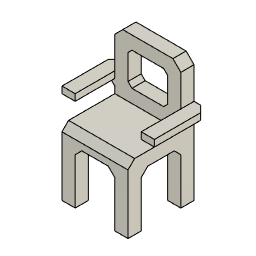
Demonstrationsmodell Kurs 3D-skrivare v3 (Autodesk Fusion 360 design; units mm, degrees)
Autodesk Fusion 360 part; units mm, degrees
sketch "Sketch1" plane through (0, 0, 0) normal (0, 0, 1) x (1, 0, 0) in component "Chair Brutaliste"
  line L0 (0, 0) -> (10, 0)
  line L1 (10, 0) -> (10, 10)
  line L2 (10, 10) -> (0, 10)
  line L3 (0, 10) -> (0, 0)
  line L4 (0, 0) -> (50, 0) construction
  line L5 (50, 0) -> (50, 50) construction
  line L6 (50, 50) -> (0, 50) construction
  line L7 (50, 0) -> (40, 0)
  line L8 (40, 0) -> (40, 10)
  line L9 (40, 10) -> (50, 10)
  line L10 (50, 10) -> (50, 0)
  line L11 (50, 50) -> (40, 50)
  line L12 (40, 50) -> (40, 40)
  line L13 (40, 40) -> (50, 40)
  line L14 (50, 40) -> (50, 50)
  line L15 (0, 50) -> (10, 50)
  line L16 (10, 50) -> (10, 40)
  line L17 (10, 40) -> (0, 40)
  line L18 (0, 40) -> (0, 50)
  dimension "d1" = 10
  dimension "d2" = 50
  constraint horizontal L0
  constraint vertical L1
  constraint horizontal L2
  constraint vertical L3
  constraint coincident L0.start L3.end
  constraint equal L1 L2
  constraint perpendicular L3 L4
  constraint perpendicular L4 L5
  constraint perpendicular L5 L6
  constraint horizontal L7
  constraint vertical L8
  constraint horizontal L9
  constraint vertical L10
  constraint horizontal L11
  constraint vertical L12
  constraint horizontal L13
  constraint vertical L14
  constraint horizontal L15
  constraint vertical L16
  constraint horizontal L17
  constraint vertical L18
  constraint equal L16 L17
  constraint equal L12 L13
  constraint equal L8 L9
  constraint equal L1 L8
  constraint equal L9 L13
  constraint equal L13 L16
  constraint equal L4 L6
  constraint equal L4 L5
  measures "d1" distance of L0.start L0.end
  measures "d2" distance of L0.start L4.end
extrude "Extrude1" add sketch "Sketch1" along normal blind 40 makes body 1 at (3.3333, 50, 13.3333) makes body 2 at (0, 6.6667, 13.3333) makes body 3 at (50, 43.3333, 13.3333) makes body 4 at (43.3333, 10, 13.3333) in component "Chair Brutaliste"
sketch "Sketch2" plane through (0, 0, 40) normal (0, 0, 1) x (-1, 0, 0) in component "Chair Brutaliste"
  line L0 (-50, -10) -> (-40, -10)
  line L1 (-40, -10) -> (-40, 0)
  line L2 (-40, 0) -> (-50, 0)
  line L3 (-50, 0) -> (-50, -10)
  line L4 (-50, -50) -> (0, -50)
  line L5 (0, -50) -> (0, 0)
  line L6 (0, 0) -> (-50, 0)
  line L7 (-50, 0) -> (-50, -50)
  constraint horizontal L4
  constraint vertical L5
  constraint horizontal L6
  constraint vertical L7
  constraint coincident L5.end L6.start
extrude "Extrude2" add sketch "Sketch2" along normal blind 10 bodies 1 2 3 4 in component "Chair Brutaliste"
sketch "Sketch3" plane through (50, 0, 0) normal (1, 0, 0) x (0, 1, 0) in component "Chair Brutaliste"
  line L0 (40, 0) -> (50, 0)
  line L1 (50, 0) -> (50, 50)
  line L2 (50, 50) -> (0, 50)
  line L3 (0, 50) -> (0, 0)
  line L4 (0, 0) -> (10, 0)
  line L5 (10, 0) -> (10, 40)
  line L6 (10, 40) -> (40, 40)
  line L7 (40, 40) -> (40, 0)
  line L8 (50, 50) -> (40, 50)
  line L9 (40, 50) -> (40, 95)
  line L10 (40, 95) -> (50, 95)
  line L11 (50, 95) -> (50, 50)
  dimension "d8" = 10
  dimension "d9" = 45
  constraint horizontal L8
  constraint vertical L9
  constraint horizontal L10
  constraint vertical L11
  constraint coincident L1.end L2.start
  measures "d8" distance of L1.end L8.end
  measures "d9" distance of L1.end L10.end
extrude "Extrude3" add sketch "Sketch3" against normal up to surface (50 mm away) contours L2 L8 L9 L10 L11 bodies 1 in component "Chair Brutaliste"
sketch "Sketch4" plane through (0, 40, 0) normal (0, -1, 0) x (1, 0, 0) in component "Chair Brutaliste"
  line L0 (0, 95) -> (0, 50)
  line L1 (0, 50) -> (50, 50)
  line L2 (50, 50) -> (50, 95)
  line L3 (50, 95) -> (0, 95)
  line L4 (10, 60) -> (40, 60)
  line L5 (40, 60) -> (40, 85)
  line L6 (40, 85) -> (10, 85)
  line L7 (10, 85) -> (10, 60)
  dimension "d13" = -10
extrude "Extrude4" cut sketch "Sketch4" against normal up to surface (10 mm away) contours L4 L5 L6 L7 bodies 1 in component "Chair Brutaliste"
chamfer "Chamfer2" distance 5 angle 45 8 edges at (10, 45, 40) (10, 5, 40) (40, 45, 40) (40, 5, 40) (5, 40, 40) (5, 10, 40) (45, 40, 40) (45, 10, 40) on bodies 1 in component "Chair Brutaliste"
chamfer "Chamfer3" distance 3 angle 45 4 edges at (40, 45, 85) (10, 45, 85) (10, 45, 60) (40, 45, 60) on bodies 1 in component "Chair Brutaliste"
chamfer "Chamfer4" distance 6 angle 45 2 edges at (50, 45, 95) (0, 45, 95) on bodies 1 in component "Chair Brutaliste"
sketch "Sketch5" plane through (50, 0, 0) normal (1, 0, 0) x (0, 1, 0) in component "Chair Brutaliste"
  line L0 (50, 89) -> (40, 89)
  line L1 (40, 89) -> (40, 50)
  line L2 (40, 50) -> (0, 50)
  line L3 (0, 50) -> (0, 0)
  line L4 (0, 0) -> (10, 0)
  line L5 (10, 0) -> (10, 35)
  line L6 (10, 35) -> (15, 40)
  line L7 (15, 40) -> (35, 40)
  line L8 (35, 40) -> (40, 35)
  line L9 (40, 35) -> (40, 0)
  line L10 (40, 0) -> (50, 0)
  line L11 (50, 0) -> (50, 89)
  line L12 (40, 50) -> (40, 60) construction
  line L13 (40, 60) -> (40, 65)
  line L14 (40, 60) -> (50, 60)
  line L15 (40, 65) -> (50, 65)
  line L16 (50, 60) -> (50, 65)
  dimension "d19" = 5
  dimension "d20" = 10
  constraint coincident L1.end L2.start
  constraint coincident L1 L12.end
  constraint perpendicular L2 L12
  constraint coincident L1 L13.end
  constraint parallel L1 L13
  constraint coincident L11 L14.end
  constraint perpendicular L11 L14
  constraint coincident L11 L15.end
  constraint perpendicular L11 L15
  measures "d19" distance of L12.end L13.end
  measures "d20" distance of L1.end L12.end
extrude "Extrude5" add sketch "Sketch5" along normal blind 10 contours L1 L11 L13 L14 L15 L16 bodies 1 in component "Chair Brutaliste"
sketch "Sketch6" plane through (0, 40, 0) normal (0, -1, 0) x (1, 0, 0) in component "Chair Brutaliste"
  line L0 (13, 85) -> (37, 85)
  line L1 (37, 85) -> (40, 82)
  line L2 (40, 82) -> (40, 63)
  line L3 (40, 63) -> (37, 60)
  line L4 (37, 60) -> (13, 60)
  line L5 (13, 60) -> (10, 63)
  line L6 (10, 63) -> (10, 82)
  line L7 (10, 82) -> (13, 85)
  line L8 (6, 95) -> (0, 89)
  line L9 (0, 89) -> (0, 50)
  line L10 (0, 50) -> (50, 50)
  line L11 (50, 50) -> (50, 60)
  line L12 (50, 60) -> (60, 60)
  line L13 (60, 60) -> (60, 65)
  line L14 (60, 65) -> (50, 65)
  line L15 (50, 65) -> (50, 89)
  line L16 (50, 89) -> (44, 95)
  line L17 (44, 95) -> (6, 95)
  line L18 (50, 65) -> (50, 60)
  constraint coincident L14.end L15.start
  constraint coincident L11.end L12.start
extrude "Extrude6" add sketch "Sketch6" along normal blind 30 contours L12 L13 L14 L18 bodies 1 in component "Chair Brutaliste"
ref_plane "WorkPlane1" through (25, 25, 44.5) normal (-1, 0, 0) x (0, -1, 0) in component "Chair Brutaliste"
mirror "Mirror1" about plane through (25, 25, 44.5) normal (-1, 0, 0) of "Extrude5" in component "Chair Brutaliste"
sketch "Sketch7" plane through (0, 40, 0) normal (0, -1, 0) x (1, 0, 0) in component "Chair Brutaliste"
  line L0 (50, 60) -> (50, 65)
  line L1 (50, 65) -> (50, 89)
  line L2 (50, 89) -> (44, 95)
  line L3 (44, 95) -> (6, 95)
  line L4 (6, 95) -> (0, 89)
  line L5 (0, 89) -> (0, 65)
  line L6 (0, 65) -> (-10, 65)
  line L7 (-10, 65) -> (-10, 60)
  line L8 (-10, 60) -> (0, 60)
  line L9 (0, 60) -> (0, 50)
  line L10 (0, 50) -> (50, 50)
  line L11 (13, 85) -> (37, 85)
  line L12 (37, 85) -> (40, 82)
  line L13 (40, 82) -> (40, 63)
  line L14 (40, 63) -> (37, 60)
  line L15 (37, 60) -> (13, 60)
  line L16 (13, 60) -> (10, 63)
  line L17 (10, 63) -> (10, 82)
  line L18 (10, 82) -> (13, 85)
  line L19 (0, 65) -> (0, 60)
  line L20 (50, 50) -> (50, 60)
  constraint coincident L5.end L6.start
  constraint coincident L8.end L9.start
extrude "Extrude7" add sketch "Sketch7" along normal up to surface (30 mm away) contours L6 L7 L8 L19 bodies 1 in component "Chair Brutaliste"
chamfer "Chamfer6" distance 5 angle 45 1 edges at (25, 0, 50) on bodies 1 in component "Chair Brutaliste"
chamfer "Chamfer7" distance 5 angle 45 2 edges at (60, 50, 62.5) (-10, 50, 62.5) on bodies 1 in component "Chair Brutaliste"
chamfer "Chamfer8" distance 5 angle 45 2 edges at (50, 45, 60) (0, 45, 60) on bodies 1 in component "Chair Brutaliste"
component "Chair Brutaliste" placed x (1, 0, 0) y (0, 1, 0) z (0, 0, 1) at (0, 0, 0)
